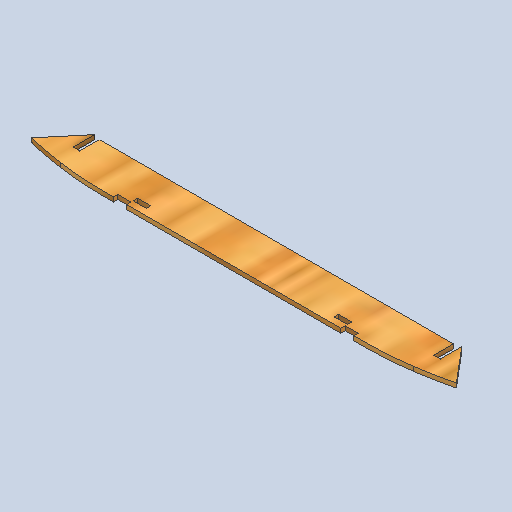
# Autodesk Inventor part: bulkhead_transom
Saved by Autodesk Inventor 2022 (Build 260153070, 153G)
## iProperties
Created: 2021-04-24
Part Number: bulkhead_transom
Material: Plywood, Sheathing, Glazed
Document SubType Name: Modeling
Designer: kardo
Density: 0.75 g/cm^3
Appearance: Plywood - New(2)
Mass: 5.0916 g
Surface Area: 77.5251 cm^2
Volume: 6.7888 cm^3
Author: kardo
Autodesk Inventor part; units mm, degrees
ref_plane "YZ Plane" through (0, 0, 0) normal (1, 0, 0) x (0, 1, 0)
ref_plane "XZ Plane" through (0, 0, 0) normal (0, 1, 0) x (-1, 0, 0)
ref_plane "XY Plane" through (0, 0, 0) normal (0, 0, 1) x (1, 0, 0)
derived "frame_parts_2_simplified.ipt"
sketch "bh_transom" plane through (0, -363, 0) normal (0, 1, 0) x (-1, 0, 0)
  line L0 (-55, 39.654) -> (0, 39.654) construction
  line L1 (-98.6155, 34.5934) -> (-81, 13.6) construction
  line L2 (-81, 13.6) -> (-81, 18.496) construction
  line L3 (-81, 18.496) -> (0, 18.496) construction
  line L4 (0, 38.854) -> (-55, 38.854)
  line L5 (-97.1793, 34.1263) -> (-81, 14.8446)
  line L6 (0, 38.854) -> (0, 19.296)
  line L7 (-81, 19.296) -> (0, 19.296)
  line L8 (-81, 14.8446) -> (-81, 19.296)
  spline S0 degree 4 poles (-81, 38.08) (-79.3784, 38.3141) (-72.9245, 39.1593) (-66.3924, 39.654) (-59.8745, 39.654) (-55, 39.654) knots 0 0 0 0 0 0.252129 1 1 1 1 1
  spline S1 degree 4 poles (-98.6155, 34.5934) (-97.3946, 34.9021) (-93.0409, 35.9563) (-88.6541, 36.856) (-84.2144, 37.616) (-81, 38.08) knots 0 0 0 0 0 0.28097 1 1 1 1 1
  spline S2 degree 3 poles (-55, 38.854) (-56.4484, 38.854) (-58.9792, 38.8536) (-61.8664, 38.8152) (-64.03, 38.7619) (-65.4714, 38.713) (-67.2719, 38.6331) (-68.7114, 38.5533) (-70.5093, 38.4329) (-71.9463, 38.3197) (-73.7407, 38.1573) (-75.1744, 38.0109) (-76.9638, 37.8084) (-78.7498, 37.5871) (-80.1745, 37.3909) (-80.8857, 37.2882) knots 0 0 0 0 0.166667 0.291667 0.333333 0.416667 0.458333 0.541667 0.583333 0.666667 0.708333 0.791667 0.833333 0.916667 1 1 1 1
  spline S3 degree 3 poles (-80.8857, 37.2882) (-81.8035, 37.1557) (-83.4063, 36.9106) (-85.2305, 36.605) (-86.5954, 36.3651) (-87.5037, 36.1999) (-88.6369, 35.9869) (-89.5418, 35.8112) (-90.671, 35.585) (-91.5727, 35.3988) (-92.6979, 35.1595) (-93.5966, 34.9627) (-94.7182, 34.71) (-95.8382, 34.4505) (-96.7325, 34.2356) (-97.1793, 34.1263) knots 0 0 0 0 0.166667 0.291667 0.333333 0.416667 0.458333 0.541667 0.583333 0.666667 0.708333 0.791667 0.833333 0.916667 1 1 1 1
  point P0 (0, 0)
  point P1 (-81, 28.288)
extrude "Extrusion1" add sketch "bh_transom" along normal blind 2
sketch "Sketch3" plane through (0, -363, 19.296) normal (0, -1, 0) x (1, 0, 0)
  line L0 (0, 19.558) -> (55, 19.558) projected
  line L1 (0, 19.558) -> (55, 19.558) projected
  line L2 (55, 19.558) -> (55, 17.558)
  line L3 (55, 17.558) -> (49, 17.558)
  line L4 (49, 14.558) -> (43, 14.558)
  line L5 (49, 17.558) -> (49, 19.558)
  line L6 (49, 14.558) -> (49, 16.558)
  line L7 (49, 16.558) -> (43, 16.558)
  line L8 (43, 14.558) -> (43, 16.558)
  line L9 (43, 16.558) -> (43, 19.558) construction
  point P0 (0, -19.296)
  point P1 (49, 19.558)
  dimension "d8" = 2
  dimension "d9" = 2
  dimension "d10" = 3
  dimension "d11" = 6
  dimension "d12" = 6
  constraints: 16 end point, 4 vertical, 3 horizontal, 3 point on line, 1 collinear
  measures "d8" distance of L4.end L7.end
  measures "d9" distance of L0.end L2.end
  measures "d10" distance of L7.end L9.end
  measures "d11" distance of L4.start L4.end
  measures "d12" distance of L2.end L3.end
sketch "Sketch2" plane through (0, -361, 19.296) normal (0, 1, 0) x (1, 0, 0)
  line L0 (81, 4.4514) -> (81, 0) projected
  line L1 (0, 0) -> (0, -19.558) projected
  line L2 (81, 0) -> (81, -8.992)
  line L3 (81, -8.992) -> (84, -8.992)
  line L4 (84, -8.992) -> (84, 4.4514)
  line L5 (84, 4.4514) -> (81, 4.4514)
  point P0 (0, 19.296)
  dimension "d3" = 19.5581
  dimension "d4" = 3
  constraints: 8 end point, 2 horizontal, 1 collinear, 1 parallel, 1 point on line
  measures "d3" distance of L1.start L1.end
  measures "d4" distance of L2.end L3.end
extrude "Extrusion2" cut sketch "Sketch2" against normal through all
extrude "Extrusion3" cut sketch "Sketch3" against normal through all
mirror "Mirror1" about plane through (0, 0, 0) normal (1, 0, 0)
equation "\"d1\" = bulkhead_thickness"
equation "\"d8\" = cowl_liner_thickness"
equation "\"d9\" = cowl_liner_thickness"
equation "\"d10\" = cowl_insulation_thickness"
equation "\"d11\" = cowl_insulation_width"
equation "\"d12\" = cowl_liner_width"
equation "\"d4\" = stringer_thickness"
equation "\"bulkhead_thickness\" = 2"
equation "\"cowl_liner_thickness\" = 2"
equation "\"cowl_insulation_thickness\" = 3"
equation "\"cowl_insulation_width\" = 6"
equation "\"cowl_liner_width\" = 6"
equation "\"stringer_thickness\" = 3"
body "Solid1"
